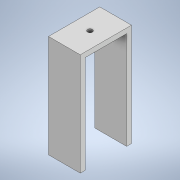
# Autodesk Inventor part: Soporteguia
Saved by Autodesk Inventor 2020 (Build 240168000, 168)
## iProperties
Created: 2019-09-28
Part Number: Soporteguia
Material: Genérico
Document SubType Name: Modeling
Designer: Java9
Density: 1 g/cm^3
Appearance: Valor por defecto
Author: Java9
Autodesk Inventor part; units mm, degrees
ref_plane "YZ Plane" through (0, 0, 0) normal (1, 0, 0) x (0, 1, 0)
ref_plane "XZ Plane" through (0, 0, 0) normal (0, 1, 0) x (-1, 0, 0)
ref_plane "XY Plane" through (0, 0, 0) normal (0, 0, 1) x (1, 0, 0)
sketch "Boceto1" plane through (0, 0, 0) normal (0, 0, 1) x (1, 0, 0)
  line L0 (0, 0) -> (130, 0)
  line L1 (130, 0) -> (130, 420)
  line L2 (130, 420) -> (0, 420)
  line L3 (0, 420) -> (0, 0)
  circle A0 centre (65, 210) radius 10
  dimension "d0" = 130
  dimension "d1" = 420
  dimension "d2" = 130
  dimension "d10" = 20
  constraints: 8 end point, 2 perpendicular, 1 centre point, 1 horizontal
  measures "d0" distance of L0.start L0.end
  measures "d1" distance of L0.end L1.end
  measures "d2" distance of L1.end L2.end
  measures "d10" diameter of A0
extrude "Extrusión1" add sketch "Boceto1" along normal blind 210 contours L3 L2 L1 L0 | A0
sketch "Boceto2" plane through (130, 0, 0) normal (1, 0, 0) x (0, 0, -1)
  line L0 (-210, 420) -> (-210, 0) projected
  line L1 (-210, 0) -> (-190, 0)
  line L2 (0, 0) -> (-210, 0) projected
  line L3 (-190, 0) -> (-190, 400)
  line L4 (-190, 400) -> (-20, 400)
  line L5 (0, 420) -> (0, 0) projected
  line L6 (-20, 400) -> (-20, 0)
  line L7 (-20, 0) -> (0, 0)
  dimension "d5" = 20
  dimension "d6" = 400
  dimension "d7" = 170
  constraints: 10 end point, 4 perpendicular, 2 point on line
  measures "d5" distance of L0.end L1.end
  measures "d6" distance of L1.end L3.end
  measures "d7" distance of L3.end L4.end
extrude "Extrusión2" cut sketch "Boceto2" against normal blind 210
sketch "Boceto3" plane through (0, 420, 0) normal (0, 1, 0) x (1, 0, 0)
  line L0 (130, 0) -> (0, 0) projected
  line L1 (130, -210) -> (0, -210) projected
  line L2 (0, 0) -> (130, -210)
  line L3 (130, 0) -> (0, -210)
  circle A0 centre (65, -105) radius 10
  dimension "d11" = 20
  constraints: 4 end point, 1 centre point, 1 midpoint
  measures "d11" diameter of A0
hole "Agujero1" at (65, 420, 105) direction (0, -1, 0) diameter 20 end through all
